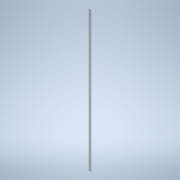
# Autodesk Inventor part: SP50V1 Acrilico Roldana
Saved by Autodesk Inventor 2021.2 (Build 252289000, 289)
## iProperties
Created: 2026-09-07
Part Number: SP50V1 Acrilico Roldana
Material: Polycarbonate, Clear
Document SubType Name: Modeling
Designer: nelso
Density: 1.2 g/cm^3
Appearance: Clear
Author: nelso
Autodesk Inventor part; units mm, degrees
ref_plane "YZ Plane" through (0, 0, 0) normal (1, 0, 0) x (0, 1, 0)
ref_plane "XZ Plane" through (0, 0, 0) normal (0, 1, 0) x (-1, 0, 0)
ref_plane "XY Plane" through (0, 0, 0) normal (0, 0, 1) x (1, 0, 0)
sketch "Sketch1" plane through (0, 0, 0) normal (0, 1, 0) x (-1, 0, 0)
  line L0 (16, 825) -> (-16, 825)
  line L1 (-16, 825) -> (-16, -825)
  line L2 (-16, -825) -> (16, -825)
  line L3 (16, -825) -> (16, 825)
  line L4 (16, 825) -> (-16, -825) construction
  line L5 (-16, 825) -> (16, -825) construction
  point P0 (0, 0)
  dimension "d0" = 32
  dimension "d1" = 1650
  constraints: 12 end point, 2 midpoint, 2 parallel, 1 horizontal, 1 perpendicular
  measures "d0" distance of L2.end L1.end
  measures "d1" distance of L1.end L0.end
extrude "Extrusion1" add sketch "Sketch1" along normal mid plane 3
sketch "Sketch2" plane through (0, 1.5, 0) normal (0, 1, 0) x (1, 0, 0)
  line L0 (16, 825) -> (-16, 825) projected
  line L1 (0, 825) -> (0, 818)
  line L2 (0, 818) -> (-10, 818)
  point P0 (0, 0)
  point P1 (10, 818)
  dimension "d4" = 7
  dimension "d5" = 10
  constraints: 4 end point, 1 coincident, 1 midpoint, 1 perpendicular, 1 symmetric about line, 1 vertical
  measures "d4" distance of L1.start L1.end
  measures "d5" distance of L1.end L2.end
hole "Hole1" at (-10, 1.5, -818) at (10, 1.5, -818) direction (0, -1, 0) diameter 3.4 end through all countersink diameter 6 countersink angle 90 clearance for "Countersunk Flat Head Screw ISO 2009/7046" size "M3" standard "ISO"
body "Solid1"
